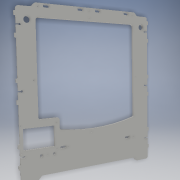
# Autodesk Inventor part: painel frontal
Saved by Autodesk Inventor 2016 (Build 200138000, 138)
## iProperties
Created: 2016-08-08
Part Number: painel frontal
Material: Generic
Document SubType Name: Modeling
Designer: Waldo
Density: 1 g/cm^3
Appearance: Default
Author: Waldo
Autodesk Inventor part; units mm, degrees
ref_plane "YZ Plane" through (0, 0, 0) normal (1, 0, 0) x (0, 1, 0)
ref_plane "XZ Plane" through (0, 0, 0) normal (0, 1, 0) x (-1, 0, 0)
ref_plane "XY Plane" through (0, 0, 0) normal (0, 0, 1) x (1, 0, 0)
sketch "Sketch1" plane through (0, 0, 0) normal (0, 1, 0) x (-1, 0, 0)
  circle A0 centre (-34.6047, -80.9896) radius 1.5
  circle A1 centre (-180.9547, 59.0104) radius 1.5
  circle A2 centre (115.8953, 59.0104) radius 1.5
  circle A3 centre (-34.6047, 213.0104) radius 1.5
  circle A4 centre (32.3863, -110.9896) radius 1.5
  circle A5 centre (103.3453, -122.3396) radius 4
  circle A6 centre (88.0953, -122.3396) radius 1.5
  circle A7 centre (70.3453, -122.3396) radius 3.5
  arc A8 (40.8953, -106.3896) -> (40.8953, -112.5896) centre (40.8953, -109.4896) ccw
  line L0 (50.8953, -106.3896) -> (40.8953, -106.3896)
  arc A9 (50.8953, -112.5896) -> (50.8953, -106.3896) centre (50.8953, -109.4896) ccw
  line L1 (40.8953, -112.5896) -> (50.8953, -112.5896)
  line L2 (67.7453, -52.9896) -> (67.7453, -104.4896)
  line L3 (146.2453, -52.9896) -> (67.7453, -52.9896)
  line L4 (146.2453, -104.4896) -> (146.2453, -52.9896)
  line L5 (67.7453, -104.4896) -> (146.2453, -104.4896)
  circle A10 centre (62.7453, -110.9896) radius 1.5
  circle A11 centre (62.7453, -45.9896) radius 1.5
  arc A12 (-155.1047, -106.3896) -> (-155.1047, -112.5896) centre (-155.1047, -109.4896) ccw
  line L6 (-145.1047, -106.3896) -> (-155.1047, -106.3896)
  arc A13 (-145.1047, -112.5896) -> (-145.1047, -106.3896) centre (-145.1047, -109.4896) ccw
  line L7 (-155.1047, -112.5896) -> (-145.1047, -112.5896)
  circle A14 centre (150.7453, -45.9896) radius 1.5
  circle A15 centre (150.7453, -110.9896) radius 1.5
  arc A16 (75.8953, 235.6104) -> (75.8953, 229.4104) centre (75.8953, 232.5104) ccw
  line L8 (85.8953, 235.6104) -> (75.8953, 235.6104)
  arc A17 (85.8953, 229.4104) -> (85.8953, 235.6104) centre (85.8953, 232.5104) ccw
  line L9 (75.8953, 229.4104) -> (85.8953, 229.4104)
  arc A18 (-155.1047, 235.6104) -> (-155.1047, 229.4104) centre (-155.1047, 232.5104) ccw
  line L10 (-145.1047, 235.6104) -> (-155.1047, 235.6104)
  arc A19 (-145.1047, 229.4104) -> (-145.1047, 235.6104) centre (-145.1047, 232.5104) ccw
  line L11 (-155.1047, 229.4104) -> (-145.1047, 229.4104)
  arc A20 (-64.6047, 235.6104) -> (-64.6047, 229.4104) centre (-64.6047, 232.5104) ccw
  line L12 (-54.6047, 235.6104) -> (-64.6047, 235.6104)
  arc A21 (-54.6047, 229.4104) -> (-54.6047, 235.6104) centre (-54.6047, 232.5104) ccw
  line L13 (-64.6047, 229.4104) -> (-54.6047, 229.4104)
  arc A22 (-14.6047, 235.6104) -> (-14.6047, 229.4104) centre (-14.6047, 232.5104) ccw
  line L14 (-4.6047, 235.6104) -> (-14.6047, 235.6104)
  arc A23 (-4.6047, 229.4104) -> (-4.6047, 235.6104) centre (-4.6047, 232.5104) ccw
  line L15 (-14.6047, 229.4104) -> (-4.6047, 229.4104)
  line L16 (153.7453, 188.8602) -> (147.2452, 188.8602)
  line L17 (153.7453, 205.76) -> (153.7453, 188.8602)
  arc A24 (155.2953, 207.31) -> (153.7453, 205.76) centre (155.2953, 205.76) ccw
  line L18 (157.8953, 207.31) -> (155.2953, 207.31)
  line L19 (157.8953, 217.3102) -> (157.8953, 207.31)
  line L20 (155.2953, 217.3102) -> (157.8953, 217.3102)
  arc A25 (153.7453, 218.8602) -> (155.2953, 217.3102) centre (155.2953, 218.8602) ccw
  line L21 (153.7453, 223.1102) -> (153.7453, 218.8602)
  arc A26 (153.7453, 223.1102) -> (147.7453, 229.1102) centre (147.7453, 223.1102) ccw
  line L22 (121.7453, 229.1102) -> (147.7453, 229.1102)
  arc A27 (115.234, 232.1465) -> (121.7453, 229.1102) centre (121.7453, 237.6102) ccw
  line L23 (112.0224, 235.9739) -> (115.234, 232.1465)
  arc A28 (112.0224, 235.9739) -> (105.511, 239.0102) centre (105.511, 230.5102) ccw
  line L24 (105.511, 239.0102) -> (-174.7203, 239.0102)
  arc A29 (-174.7203, 239.0102) -> (-181.2317, 235.9739) centre (-174.7203, 230.5102) ccw
  line L25 (-181.2317, 235.9739) -> (-184.4433, 232.1465)
  arc A30 (-190.9547, 229.1102) -> (-184.4433, 232.1465) centre (-190.9547, 237.6102) ccw
  line L26 (-190.9547, 229.1102) -> (-216.9547, 229.1102)
  arc A31 (-216.9547, 229.1102) -> (-222.9547, 223.1102) centre (-216.9547, 223.1102) ccw
  line L27 (-222.9547, 223.1102) -> (-222.9547, 218.8602)
  arc A32 (-224.5047, 217.3102) -> (-222.9547, 218.8602) centre (-224.5047, 218.8602) ccw
  line L28 (-224.5047, 217.3102) -> (-227.1047, 217.3102)
  line L29 (-227.1047, 217.3102) -> (-227.1047, 207.31)
  line L30 (-227.1047, 207.31) -> (-224.5047, 207.31)
  arc A33 (-222.9547, 205.76) -> (-224.5047, 207.31) centre (-224.5047, 205.76) ccw
  line L31 (-222.9547, 205.76) -> (-222.9547, 188.8602)
  line L32 (-216.4542, 188.8602) -> (-222.9547, 188.8602)
  arc A34 (-214.9443, 190.0602) -> (-216.4542, 188.8602) centre (-214.9443, 188.5102) ccw
  line L33 (-213.3943, 190.0602) -> (-214.9443, 190.0602)
  arc A35 (-211.8812, 188.8463) -> (-213.3943, 190.0602) centre (-213.3943, 188.5102) ccw
  line L34 (-211.8812, 188.6772) -> (-211.8812, 188.8463)
  arc A36 (-211.8812, 185.9432) -> (-211.8812, 188.6772) centre (-212.6117, 187.3102) ccw
  line L35 (-211.8812, 185.7741) -> (-211.8812, 185.9432)
  arc A37 (-213.3943, 184.5602) -> (-211.8812, 185.7741) centre (-213.3943, 186.1102) ccw
  line L36 (-214.9443, 184.5602) -> (-213.3943, 184.5602)
  arc A38 (-216.4542, 185.7602) -> (-214.9443, 184.5602) centre (-214.9443, 186.1102) ccw
  line L37 (-222.9547, 185.7602) -> (-216.4542, 185.7602)
  line L38 (-222.9547, 185.7602) -> (-222.9547, 168.8609)
  arc A39 (-224.5047, 167.3109) -> (-222.9547, 168.8609) centre (-224.5047, 168.8609) ccw
  line L39 (-227.1047, 167.3109) -> (-224.5047, 167.3109)
  line L40 (-227.1047, 157.3113) -> (-227.1047, 167.3109)
  line L41 (-224.5047, 157.3113) -> (-227.1047, 157.3113)
  arc A40 (-222.9547, 155.7613) -> (-224.5047, 157.3113) centre (-224.5047, 155.7613) ccw
  line L42 (-222.9547, 155.7613) -> (-222.9547, 65.5606)
  arc A41 (-224.5047, 64.0106) -> (-222.9547, 65.5606) centre (-224.5047, 65.5606) ccw
  line L43 (-224.5047, 64.0106) -> (-227.1047, 64.0106)
  line L44 (-227.1047, 64.0106) -> (-227.1047, 54.0109)
  line L45 (-227.1047, 54.0109) -> (-224.5047, 54.0109)
  arc A42 (-222.9547, 52.4609) -> (-224.5047, 54.0109) centre (-224.5047, 52.4609) ccw
  line L46 (-222.9547, 35.5609) -> (-222.9547, 52.4609)
  line L47 (-216.4544, 35.5609) -> (-222.9547, 35.5609)
  arc A43 (-214.9445, 36.7609) -> (-216.4544, 35.5609) centre (-214.9445, 35.2109) ccw
  line L48 (-213.3945, 36.7609) -> (-214.9445, 36.7609)
  arc A44 (-211.8813, 35.547) -> (-213.3945, 36.7609) centre (-213.3945, 35.2109) ccw
  line L49 (-211.8813, 35.3779) -> (-211.8813, 35.547)
  arc A45 (-211.8813, 32.6439) -> (-211.8813, 35.3779) centre (-212.6119, 34.0109) ccw
  line L50 (-211.8813, 32.4748) -> (-211.8813, 32.6439)
  arc A46 (-213.3945, 31.2609) -> (-211.8813, 32.4748) centre (-213.3945, 32.8109) ccw
  line L51 (-214.9445, 31.2609) -> (-213.3945, 31.2609)
  arc A47 (-216.4544, 32.4609) -> (-214.9445, 31.2609) centre (-214.9445, 32.8109) ccw
  line L52 (-222.9547, 32.4609) -> (-216.4544, 32.4609)
  line L53 (-222.9547, 15.5606) -> (-222.9547, 32.4609)
  arc A48 (-224.5047, 14.0106) -> (-222.9547, 15.5606) centre (-224.5047, 15.5606) ccw
  line L54 (-227.1047, 14.0106) -> (-224.5047, 14.0106)
  line L55 (-227.1047, 4.0106) -> (-227.1047, 14.0106)
  line L56 (-224.5047, 4.0106) -> (-227.1047, 4.0106)
  arc A49 (-222.9547, 2.4606) -> (-224.5047, 4.0106) centre (-224.5047, 2.4606) ccw
  line L57 (-222.9547, -87.7394) -> (-222.9547, 2.4606)
  arc A50 (-224.5047, -89.2894) -> (-222.9547, -87.7394) centre (-224.5047, -87.7394) ccw
  line L58 (-224.5047, -89.2894) -> (-227.1047, -89.2894)
  line L59 (-227.1047, -89.2894) -> (-227.1047, -99.2894)
  line L60 (-227.1047, -99.2894) -> (-224.5047, -99.2894)
  arc A51 (-222.9547, -100.8394) -> (-224.5047, -99.2894) centre (-224.5047, -100.8394) ccw
  line L61 (-222.9547, -117.7396) -> (-222.9547, -100.8394)
  line L62 (-216.4544, -117.7396) -> (-222.9547, -117.7396)
  arc A52 (-214.9445, -116.5396) -> (-216.4544, -117.7396) centre (-214.9445, -118.0896) ccw
  line L63 (-213.3945, -116.5396) -> (-214.9445, -116.5396)
  arc A53 (-211.8813, -117.7535) -> (-213.3945, -116.5396) centre (-213.3945, -118.0896) ccw
  line L64 (-211.8813, -117.9226) -> (-211.8813, -117.7535)
  arc A54 (-211.8813, -120.6566) -> (-211.8813, -117.9226) centre (-212.6119, -119.2896) ccw
  line L65 (-211.8813, -120.8259) -> (-211.8813, -120.6566)
  arc A55 (-213.3944, -122.0396) -> (-211.8813, -120.8259) centre (-213.3944, -120.4896) ccw
  line L66 (-214.9445, -122.0396) -> (-213.3944, -122.0396)
  arc A56 (-216.4544, -120.8396) -> (-214.9445, -122.0396) centre (-214.9445, -120.4896) ccw
  line L67 (-222.9547, -120.8396) -> (-216.4544, -120.8396)
  line L68 (-222.9547, -137.7398) -> (-222.9547, -120.8396)
  arc A57 (-224.5047, -139.2898) -> (-222.9547, -137.7398) centre (-224.5047, -137.7398) ccw
  line L69 (-227.1047, -139.2898) -> (-224.5047, -139.2898)
  line L70 (-227.1047, -149.2898) -> (-227.1047, -139.2898)
  line L71 (-224.5047, -149.2898) -> (-227.1047, -149.2898)
  arc A58 (-222.9547, -150.8398) -> (-224.5047, -149.2898) centre (-224.5047, -150.8398) ccw
  line L72 (-222.9547, -150.8398) -> (-222.9547, -174.9898)
  arc A59 (-222.9547, -174.9898) -> (-216.9547, -180.9898) centre (-216.9547, -174.9898) ccw
  line L73 (-216.9547, -180.9898) -> (-184.9547, -180.9898)
  arc A60 (-184.9547, -180.9898) -> (-178.4433, -177.9535) centre (-184.9547, -172.4898) ccw
  line L74 (-178.4433, -177.9535) -> (-174.2511, -172.9575)
  arc A61 (-170.0314, -170.9898) -> (-174.2511, -172.9575) centre (-170.0314, -176.4982) ccw
  line L75 (100.8221, -170.9898) -> (-170.0314, -170.9898)
  arc A62 (105.0418, -172.9575) -> (100.8221, -170.9898) centre (100.8221, -176.4982) ccw
  line L76 (109.234, -177.9535) -> (105.0418, -172.9575)
  arc A63 (109.234, -177.9535) -> (115.7453, -180.9898) centre (115.7453, -172.4898) ccw
  line L77 (147.7453, -180.9898) -> (115.7453, -180.9898)
  arc A64 (147.7453, -180.9898) -> (153.7453, -174.9898) centre (147.7453, -174.9898) ccw
  line L78 (153.7453, -150.8398) -> (153.7453, -174.9898)
  arc A65 (155.2953, -149.2898) -> (153.7453, -150.8398) centre (155.2953, -150.8398) ccw
  line L79 (155.2953, -149.2898) -> (157.8953, -149.2898)
  line L80 (157.8953, -149.2898) -> (157.8953, -139.2898)
  line L81 (157.8953, -139.2898) -> (155.2953, -139.2898)
  arc A66 (153.7453, -137.7398) -> (155.2953, -139.2898) centre (155.2953, -137.7398) ccw
  line L82 (153.7453, -137.7398) -> (153.7453, -120.8396)
  line L83 (147.2451, -120.8396) -> (153.7453, -120.8396)
  arc A67 (145.7352, -122.0396) -> (147.2451, -120.8396) centre (145.7352, -120.4896) ccw
  line L84 (144.1851, -122.0396) -> (145.7352, -122.0396)
  arc A68 (142.672, -120.8259) -> (144.1851, -122.0396) centre (144.1851, -120.4896) ccw
  line L85 (142.672, -120.6566) -> (142.672, -120.8259)
  arc A69 (142.672, -117.9226) -> (142.672, -120.6566) centre (143.4026, -119.2896) ccw
  line L86 (142.672, -117.7535) -> (142.672, -117.9226)
  arc A70 (144.1852, -116.5396) -> (142.672, -117.7535) centre (144.1852, -118.0896) ccw
  line L87 (145.7352, -116.5396) -> (144.1852, -116.5396)
  arc A71 (147.2451, -117.7396) -> (145.7352, -116.5396) centre (145.7352, -118.0896) ccw
  line L88 (153.7453, -117.7396) -> (147.2451, -117.7396)
  line L89 (153.7453, -117.7396) -> (153.7453, -100.8394)
  arc A72 (155.2953, -99.2894) -> (153.7453, -100.8394) centre (155.2953, -100.8394) ccw
  line L90 (157.8953, -99.2894) -> (155.2953, -99.2894)
  line L91 (157.8953, -89.2894) -> (157.8953, -99.2894)
  line L92 (155.2953, -89.2894) -> (157.8953, -89.2894)
  arc A73 (153.7453, -87.7394) -> (155.2953, -89.2894) centre (155.2953, -87.7394) ccw
  line L93 (153.7453, -87.7394) -> (153.7453, 2.4606)
  arc A74 (155.2953, 4.0106) -> (153.7453, 2.4606) centre (155.2953, 2.4606) ccw
  line L94 (155.2953, 4.0106) -> (157.8953, 4.0106)
  line L95 (157.8953, 4.0106) -> (157.8953, 14.0106)
  line L96 (157.8953, 14.0106) -> (155.2953, 14.0106)
  arc A75 (153.7453, 15.5606) -> (155.2953, 14.0106) centre (155.2953, 15.5606) ccw
  line L97 (153.7453, 15.5606) -> (153.7453, 32.4609)
  line L98 (147.2451, 32.4609) -> (153.7453, 32.4609)
  arc A76 (145.7352, 31.2609) -> (147.2451, 32.4609) centre (145.7352, 32.8109) ccw
  line L99 (144.1852, 31.2609) -> (145.7352, 31.2609)
  arc A77 (142.672, 32.4748) -> (144.1852, 31.2609) centre (144.1852, 32.8109) ccw
  line L100 (142.672, 32.6439) -> (142.672, 32.4748)
  arc A78 (142.672, 35.3779) -> (142.672, 32.6439) centre (143.4026, 34.0109) ccw
  line L101 (142.672, 35.547) -> (142.672, 35.3779)
  arc A79 (144.1852, 36.7609) -> (142.672, 35.547) centre (144.1852, 35.2109) ccw
  line L102 (145.7352, 36.7609) -> (144.1852, 36.7609)
  arc A80 (147.2451, 35.5609) -> (145.7352, 36.7609) centre (145.7352, 35.2109) ccw
  line L103 (153.7453, 35.5609) -> (147.2451, 35.5609)
  line L104 (153.7453, 35.5609) -> (153.7453, 52.4609)
  arc A81 (155.2953, 54.0109) -> (153.7453, 52.4609) centre (155.2953, 52.4609) ccw
  line L105 (157.8953, 54.0109) -> (155.2953, 54.0109)
  line L106 (157.8953, 64.0106) -> (157.8953, 54.0109)
  line L107 (155.2953, 64.0106) -> (157.8953, 64.0106)
  arc A82 (153.7453, 65.5606) -> (155.2953, 64.0106) centre (155.2953, 65.5606) ccw
  line L108 (153.7453, 155.7613) -> (153.7453, 65.5606)
  arc A83 (155.2953, 157.3113) -> (153.7453, 155.7613) centre (155.2953, 155.7613) ccw
  line L109 (155.2953, 157.3113) -> (157.8953, 157.3113)
  line L110 (157.8953, 157.3113) -> (157.8953, 167.3109)
  line L111 (157.8953, 167.3109) -> (155.2953, 167.3109)
  arc A84 (153.7453, 168.8609) -> (155.2953, 167.3109) centre (155.2953, 168.8609) ccw
  line L112 (153.7453, 185.7602) -> (153.7453, 168.8609)
  line L113 (147.2451, 185.7602) -> (153.7453, 185.7602)
  arc A85 (145.7352, 184.5602) -> (147.2451, 185.7602) centre (145.7352, 186.1102) ccw
  line L114 (144.1852, 184.5602) -> (145.7352, 184.5602)
  arc A86 (142.672, 185.7741) -> (144.1852, 184.5602) centre (144.1852, 186.1102) ccw
  line L115 (142.672, 185.9432) -> (142.672, 185.7741)
  arc A87 (142.672, 188.6772) -> (142.672, 185.9432) centre (143.4026, 187.3102) ccw
  line L116 (142.672, 188.8463) -> (142.672, 188.6772)
  arc A88 (144.1852, 190.0602) -> (142.672, 188.8463) centre (144.1852, 188.5102) ccw
  line L117 (145.7352, 190.0602) -> (144.1852, 190.0602)
  arc A89 (147.2452, 188.8602) -> (145.7352, 190.0602) centre (145.7352, 188.5102) ccw
  circle A90 centre (-201.1047, 198.6104) radius 8
  circle A91 centre (128.7453, 198.6104) radius 8
  circle A92 centre (-170.9547, -110.9896) radius 1.6
  circle A93 centre (-170.9547, 231.0104) radius 1.6
  circle A94 centre (101.7453, 231.0104) radius 1.6
  line L118 (103.8764, -34.1419) -> (58.9808, -34.1419)
  arc A95 (58.9808, -34.1419) -> (54.0552, -39.0675) centre (58.9808, -39.0675) ccw
  line L119 (54.0552, -39.0675) -> (54.0552, -60.8574)
  arc A96 (50.2783, -65.2775) -> (54.0552, -60.8574) centre (49.5804, -60.8574) ccw
  arc A97 (-169.9156, -53.6221) -> (50.2783, -65.2775) centre (-32.4058, 458.4336) ccw
  arc A98 (-172.9545, -49.6594) -> (-169.9156, -53.6221) centre (-168.8514, -49.6594) ccw
  line L120 (-172.9545, 198.511) -> (-172.9545, -49.6594)
  arc A99 (-166.4545, 205.011) -> (-172.9545, 198.511) centre (-166.4545, 198.511) ccw
  line L121 (101.3955, 205.011) -> (-166.4545, 205.011)
  arc A100 (107.8955, 198.511) -> (101.3955, 205.011) centre (101.3955, 198.511) ccw
  line L122 (107.8955, -30.1228) -> (107.8955, 198.511)
  arc A101 (103.8764, -34.1419) -> (107.8955, -30.1228) centre (103.8764, -30.1228) ccw
  circle A102 centre (-34.6047, 231.0104) radius 1.6
  point P0 (0, 0)
  constraints: 246 end point, 232 tangent, 170 point on circle, 103 centre point, 87 equal radius, 64 parallel, 11 perpendicular, 1 collinear
extrude "Extrusion1" add sketch "Sketch1" along normal blind 6
body "Solid1"
